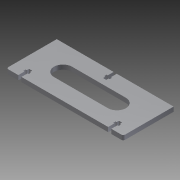
# Autodesk Inventor part: pieza protectora 2
Saved by Autodesk Inventor 2012 (Build 160160000, 160)
## iProperties
Created: 2014-12-16
Part Number: pieza protectora 2
Material: Default
Document SubType Name: Modeling
Designer: PRINCIPAL
Density: 1 g/cm^3
Author: PRINCIPAL
Autodesk Inventor part; units mm, degrees
ref_plane "YZ Plane" through (0, 0, 0) normal (1, 0, 0) x (0, 1, 0)
ref_plane "XZ Plane" through (0, 0, 0) normal (0, 1, 0) x (-1, 0, 0)
ref_plane "XY Plane" through (0, 0, 0) normal (0, 0, 1) x (1, 0, 0)
sketch "Boceto1" plane through (0, 0, 0) normal (0, 0, 1) x (1, 0, 0)
  line L0 (0, 0) -> (130, 0)
  line L1 (130, 0) -> (130, -56.08)
  line L2 (130, -56.08) -> (0, -56.08)
  line L3 (0, -56.08) -> (0, 0)
  dimension "d0" = 130
  dimension "d1" = 56.08
  constraints: 8 end point, 2 parallel, 1 horizontal, 1 perpendicular
  measures "d0" distance of L1.end L2.end
  measures "d1" distance of L0.end L1.end
extrude "Extrusión1" add sketch "Boceto1" along normal blind 5
sketch "Boceto2" plane through (0, 0, 5) normal (0, 0, 1) x (1, 0, 0)
  line L0 (130, 0) -> (130, -56.08) projected
  line L1 (0, -56.08) -> (0, 0) projected
  line L2 (130, -56.08) -> (0, -56.08) projected
  line L3 (16.75, -57.2435) -> (13.25, -57.2435)
  line L4 (13.25, -44.08) -> (16.75, -44.08)
  line L5 (116.75, -57.2435) -> (113.25, -57.2435)
  line L6 (113.25, -44.08) -> (116.75, -44.08)
  line L7 (12, -46.6661) -> (12, -49.2661)
  line L8 (18, -49.2661) -> (18, -46.6661)
  line L9 (112, -46.6661) -> (112, -49.2661)
  line L10 (118, -49.2661) -> (118, -46.6661)
  line L11 (12, -49.2661) -> (13.25, -49.2661)
  line L12 (16.75, -49.2661) -> (18, -49.2661)
  line L13 (16.75, -44.08) -> (16.75, -46.6661)
  line L14 (16.75, -49.2661) -> (16.75, -57.2435)
  line L15 (18, -46.6661) -> (16.75, -46.6661)
  line L16 (13.25, -46.6661) -> (12, -46.6661)
  line L17 (13.25, -57.2435) -> (13.25, -49.2661)
  line L18 (13.25, -46.6661) -> (13.25, -44.08)
  line L19 (112, -49.2661) -> (113.25, -49.2661)
  line L20 (116.75, -49.2661) -> (118, -49.2661)
  line L21 (116.75, -44.08) -> (116.75, -46.6661)
  line L22 (116.75, -49.2661) -> (116.75, -57.2435)
  line L23 (118, -46.6661) -> (116.75, -46.6661)
  line L24 (113.25, -46.6661) -> (112, -46.6661)
  line L25 (113.25, -57.2435) -> (113.25, -49.2661)
  line L26 (113.25, -46.6661) -> (113.25, -44.08)
  dimension "d7" = 6
  dimension "d8" = 12
  dimension "d14" = 13.25
  dimension "d15" = 1.25
  dimension "d16" = 1.25
  dimension "d17" = 13.25
  dimension "d18" = 3.5
  constraints: 48 end point, 20 parallel, 8 perpendicular, 6 horizontal
  measures "d7" distance between parallel lines of L10 L9
  measures "d8" distance between parallel lines of L6 L2
  measures "d14" distance between parallel lines of L1 L17
  measures "d15" distance between parallel lines of L7 L18
  measures "d16" distance between parallel lines of L10 L21
  measures "d17" distance between parallel lines of L0 L22
  measures "d18" distance between parallel lines of L22 L25
extrude "Extrusión2" cut sketch "Boceto2" against normal blind 5
sketch "Boceto3" plane through (0, 0, 5) normal (0, 0, 1) x (1, 0, 0)
  line L0 (0, -56.08) -> (0, 0) projected
  line L1 (63.25, -6.5636) -> (63.25, 0.2503)
  line L2 (66.75, 0.2503) -> (66.75, -6.5636)
  line L3 (66.75, -6.5636) -> (68, -6.5636)
  line L4 (68, -6.5636) -> (68, -9.1636)
  line L5 (68, -9.1636) -> (66.75, -9.1636)
  line L6 (66.75, -9.1636) -> (66.75, -11.7497)
  line L7 (66.75, -11.7497) -> (63.25, -11.7497)
  line L8 (63.25, -11.7497) -> (63.25, -9.1636)
  line L9 (63.25, -9.1636) -> (62, -9.1636)
  line L10 (62, -9.1636) -> (62, -6.5636)
  line L11 (62, -6.5636) -> (63.25, -6.5636)
  line L12 (63.25, 0.2503) -> (66.75, 0.2503)
  dimension "d21" = 63.25
  constraints: 24 end point, 1 perpendicular
  measures "d21" distance between parallel lines of L0 L1
extrude "Extrusión3" cut sketch "Boceto3" against normal blind 5
fillet "Empalme1" radius 2 1 edges at (130, -56.08, 2.5)
fillet "Empalme2" radius 2 1 edges at (0, -56.08, 2.5)
sketch "Boceto4" plane through (0, 0, 5) normal (0, 0, 1) x (1, 0, 0)
  line L0 (113.25, -56.08) -> (16.75, -56.08) projected
  line L1 (0, -54.08) -> (0, 0) projected
  arc A0 (35, -18.08) -> (35, -38.08) centre (35, -28.08) ccw
  arc A1 (95, -38.08) -> (95, -18.08) centre (95, -28.08) ccw
  line L2 (35, -38.08) -> (95, -38.08)
  line L3 (95, -18.08) -> (35, -18.08)
  dimension "d26" = 20
  dimension "d27" = 20
  dimension "d28" = 60
  dimension "d29" = 35
  dimension "d30" = 28
  constraints: 4 end point, 4 point on circle, 3 tangent, 2 centre point, 1 perpendicular
  measures "d26" diameter of A0
  measures "d27" diameter of A1
  measures "d28" distance of A1.centre A0.centre
  measures "d29" distance from line of L1 A0.centre
  measures "d30" distance from line of L0 A0.centre
extrude "Extrusión4" cut sketch "Boceto4" against normal blind 5
